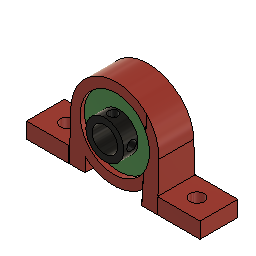
BEARING BLOCK (Autodesk Fusion 360 design; units mm, degrees)
Autodesk Fusion 360 part; units mm, degrees
sketch "Sketch1" plane through (0, 0, 0) normal (0, 1, 0) x (1, 0, 0)
  circle A0 centre (0, 0) radius 11
  circle A1 centre (0, 0) radius 14
  line L0 (14, 0) -> (14, 10)
  line L1 (14, 10) -> (27.5, 10)
  line L2 (27.5, 10) -> (27.5, 15)
  line L3 (27.5, 15) -> (9, 15)
  line L4 (9, 15) -> (9, 10.7238)
  line L5 (0, -18.3695) -> (0, 20.4506)
  line L6 (-14, 10) -> (-27.5, 10)
  line L7 (-14, 0) -> (-14, 10)
  line L8 (-9, 15) -> (-9, 10.7238)
  line L9 (-27.5, 10) -> (-27.5, 15)
  line L10 (-27.5, 15) -> (-9, 15)
  dimension "d1" = 22
  dimension "d2" = 28
  dimension "d3" = 10
  dimension "d4" = 13.5
  dimension "d5" = 5
  dimension "d6" = 18.5
  constraint coincident A0.centre A1.centre
  constraint concentric A0 A1
  constraint coincident A1 L0.start
  constraint vertical L0
  constraint perpendicular L0 L1
  constraint perpendicular L1 L2
  constraint perpendicular L2 L3
  constraint perpendicular L3 L4
  constraint vertical L5
  constraint coincident A1 L4.end
  constraint tangent A1 L0
  constraint symmetric L0.start L5 L7.start
  constraint symmetric L0.end L5 L6.start
  constraint symmetric L1.end L5 L6.end
  constraint symmetric L2.end L5 L9.end
  constraint symmetric L3.end L5 L8.start
  constraint symmetric L4.end L5 L8.end
  measures "d1" diameter of A0
  measures "d2" diameter of A1
  measures "d3" distance of L0.start L0.end
  measures "d4" distance of L0.end L1.end
  measures "d5" distance of L1.end L2.end
  measures "d6" distance of L2.end L3.end
extrude "Extrude1" add sketch "Sketch1" along normal mid plane 12 contours A0 A1 L5 | A0 A1 L5 | A1 L0 L1 L2 L3 L4 | A1 L6 L7 L8 L9 L10 makes body 1
sketch "Sketch3" plane through (0, 0, -15) normal (0, 0, -1) x (1, 0, 0)
  line L0 (-27.5, 6) -> (-27.5, -6)
  line L1 (-27.5, -6) -> (-9, -6)
  line L2 (-9, -6) -> (-9, 6)
  line L3 (-9, 6) -> (-27.5, 6)
  line L4 (14.0403, 5.9533) -> (-13.9519, 5.9533)
  line L5 (-13.9519, 5.9533) -> (-13.9519, 6.3706)
  line L6 (-13.9519, 6.3706) -> (14.0403, 6.3706)
  line L7 (14.0403, 6.3706) -> (14.0403, 5.9533)
  line L8 (14.0082, 0) -> (-13.7914, 0)
  line L9 (14.0403, -5.9533) -> (-13.9519, -5.9533)
  line L10 (-13.9519, -6.3706) -> (14.0403, -6.3706)
  line L11 (-13.9519, -5.9533) -> (-13.9519, -6.3706)
  line L12 (14.0403, -6.3706) -> (14.0403, -5.9533)
  point P0 (-9, -6)
  constraint horizontal L4
  constraint vertical L5
  constraint horizontal L6
  constraint vertical L7
  constraint perpendicular L2 L8
  constraint symmetric L2.end L8 P0
  constraint symmetric L4.start L8 L9.start
  constraint symmetric L4.end L8 L9.end
  constraint symmetric L5.end L8 L10.start
  constraint symmetric L6.end L8 L10.end
extrude "Extrude3" cut sketch "Sketch3" against normal blind 35 draft 1.8 contours L2 L3 L4 L5 L6 L7 | L1 L2 L9 L10 L11 L12 bodies 1
sketch "Sketch4" plane through (0, 0, 0) normal (0, 1, 0) x (1, 0, 0)
  circle A0 centre (0, 0) radius 11
  circle A1 centre (0, 0) radius 6
  dimension "d13" = 22
  dimension "d14" = 12
  constraint coincident A0.centre A1.centre
  measures "d13" diameter of A0
  measures "d14" diameter of A1
extrude "Extrude4" add sketch "Sketch4" along normal mid plane 7 separate body makes body 2
sketch "Sketch5" plane through (0, 0, 0) normal (0, 1, 0) x (1, 0, 0)
  circle A0 centre (0, 0) radius 6
  circle A1 centre (0, 0) radius 4
  dimension "d17" = 12
  dimension "d18" = 8
  constraint coincident A0.centre A1.centre
  constraint concentric A0 A1
  measures "d17" diameter of A0
  measures "d18" diameter of A1
extrude "Extrude5" add sketch "Sketch5" along normal blind 11.5 from surface at -3.5 separate body makes body 3
ref_plane "WorkPlane1" through (0, 5.3931, 6) normal (0, 0, 1) x (-1, 0, 0)
sketch "Sketch6" plane through (0, 0, 6) normal (0, 0, 1) x (1, 0, 0)
  circle A0 centre (0, 5.5) radius 1.5
  line L0 (6, 8) -> (-6, 8)
  dimension "d23" = 3
  dimension "d27" = 2.5
  measures "d23" diameter of A0
  measures "d27" distance of A0.centre L0
ref_plane "WorkPlane2" through (-6, 4.2384, 0) normal (-1, 0, 0) x (0, 0, -1)
sketch "Sketch7" plane through (-6, 0, 0) normal (-1, 0, 0) x (0, -1, 0)
  circle A0 centre (-5.5, 0) radius 1.5
  point P0 (-8, 0)
  dimension "d25" = 3
  dimension "d26" = 2.5
  measures "d25" diameter of A0
  measures "d26" distance of A0.centre P0
extrude "Extrude6" cut sketch "Sketch6" against normal blind 3 bodies 3
extrude "Extrude7" cut sketch "Sketch7" against normal blind 5 bodies 3
sketch "Sketch8" plane through (0, 0, -15) normal (0, 0, -1) x (1, 0, 0)
  line L0 (9, -5.9533) -> (14.0403, -5.9533)
  line L1 (14.0403, -5.9533) -> (14.0403, -6)
  line L2 (14.0403, -6) -> (27.5, -6)
  line L3 (27.5, -6) -> (27.5, 6)
  line L4 (27.5, 6) -> (14.0403, 6)
  line L5 (14.0403, 6) -> (14.0403, 5.9533)
  line L6 (14.0403, 5.9533) -> (9, 5.9533)
  line L7 (9, 5.9533) -> (9, -5.9533)
  circle A0 centre (20.5, 0) radius 2.25
  line L8 (-0.0396, -10.534) -> (-0.0396, 12.1162)
  circle A1 centre (-20.5793, 0) radius 2.25
  dimension "d32" = 4.5
  dimension "d33" = 7
  constraint vertical L8
  constraint symmetric A0 L8 A1
  measures "d32" diameter of A0
  measures "d33" distance of L3 A0.centre
extrude "Extrude8" cut sketch "Sketch8" against normal blind 13 contours A0 | A1 bodies 1
copy_body "Body->Comp1" bodies 1 removing the originals makes body 4 in component "HOUSING"
copy_body "Body->Comp2" bodies 2 removing the originals makes body 5 in component "BEARING"
copy_body "Body->Comp3" bodies 3 removing the originals makes body 6 in component "ROTOR"
move_body "Move1" bodies 6 to x (1, 0, 0) y (0, 1, 0) z (0, 0, 1) at (0, 25, 0) in component "ROTOR"
move_body "Move1'" bodies 5 to x (1, 0, 0) y (0, 1, 0) z (0, 0, 1) at (0, -20, 0) in component "BEARING"
move_body "Move1''" bodies 4 to x (-1, 0, 0) y (0, -1, 0) z (0, 0, 1) at (-12.0028, -5.6553, 0) in component "HOUSING"
move_body "Move2" bodies 5 to x (-1, 0, 0) y (0, -1, 0) z (0, 0, 1) at (-12.0028, -47, 0) in component "BEARING"
move_body "Move2'" bodies 6 to x (-1, 0, 0) y (0, -1, 0) z (0, 0, 1) at (-12.0028, 43, 0) in component "ROTOR"
component "BEARING" placed x (1, 0, 0) y (0, 1, 0) z (0, 0, 1) at (0, 20.6724, 0)
component "ROTOR" placed x (1, 0, 0) y (0, 1, 0) z (0, 0, 1) at (0, -24.3276, 0)
component "HOUSING" placed x (1, 0, 0) y (0, 1, 0) z (0, 0, 1) at (0, 0, 0)
named bodies: "HOUSING", "BEARING", "ROTOR"
